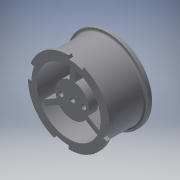
# Autodesk Inventor part: Wheel
Saved by Autodesk Inventor 2018 (Build 220112000, 112)
## iProperties
Created: 2018-12-29
Part Number: Wheel
Material: Типовые
Document SubType Name: Modeling
Designer: kostya
Density: 1 g/cm^3
Appearance: По умолчанию
Mass: 14.1359 g
Surface Area: 114.786 cm^2
Volume: 14.1359 cm^3
Author: kostya
Autodesk Inventor part; units mm, degrees
ref_plane "YZ Plane" through (0, 0, 0) normal (1, 0, 0) x (0, 1, 0)
ref_plane "XZ Plane" through (0, 0, 0) normal (0, 1, 0) x (-1, 0, 0)
ref_plane "XY Plane" through (0, 0, 0) normal (0, 0, 1) x (1, 0, 0)
sketch "Эскиз1" plane through (0, 0, 0) normal (0, 0, 1) x (1, 0, 0)
  line L0 (0, 0) -> (18, 0) construction
  line L1 (18, 0) -> (18, 24)
  line L2 (18, 24) -> (23, 24)
  line L3 (23, 0) -> (23, 24)
  line L4 (18, 0) -> (23, 0)
  line L5 (0, -4.8) -> (0, 28.8) projected
  line L6 (23, 0) -> (23, 2)
  line L7 (23, 2) -> (21, 2) construction
  line L8 (21, 3) -> (21, 18)
  line L9 (23, 24) -> (23, 22) construction
  line L10 (23, 22) -> (22, 22)
  line L11 (21, 21) -> (21, 18)
  arc A0 (22, 22) -> (21, 21) centre (22, 21) ccw
  line L12 (23, 12) -> (21, 12) construction
  arc A1 (21, 3) -> (22, 2) centre (22, 3) ccw
  line L13 (23, 2) -> (22, 2)
  point P0 (23, 18)
  dimension "d0" = 18
  dimension "d1" = 24
  dimension "d2" = 5
  dimension "d21" = 2
  dimension "d22" = 2
  dimension "d46" = 2
  constraints: 26 end point, 6 perpendicular, 4 point on circle, 4 point on line, 3 horizontal, 3 symmetric about line, 3 tangent, 2 centre point, 1 midpoint, 1 vertical, 1 other
  measures "d0" distance of L0.start L0.end
  measures "d1" distance of L0.end L1.end
  measures "d2" distance of L1.end L2.end
  measures "d21" distance of L3.start L6.end
  measures "d22" distance of L6.end L7.end
  measures "d46" distance of L2.end L9.end
revolve "Вращение1" add sketch "Эскиз1" angle 360 about axis through (0, -10, 0) along (0, 1, 0) contours L1 L2 L3 L10 A0 L11 L8 A1 L13 L4
ref_plane "РабПлоскость1" through (0, 12, 0) normal (0, 1, 0) x (1, 0, 0)
sketch "Эскиз5" plane through (0, 12, 0) normal (0, 1, 0) x (1, 0, 0)
  arc A0 (-1.0954, 0.95) -> (1.0954, 0.95) centre (0, 0) ccw
  line L0 (0.0475, -1.9475) -> (0.0475, 0.4525)
  line L1 (-1.0954, 0.95) -> (1.0954, 0.95)
  circle A1 centre (0, 0) radius 3
  circle A2 centre (0, 0) radius 18 projected
  circle A3 centre (0, 0) radius 18 projected
  line L2 (0.1379, -2.9968) -> (1.4256, -17.9435) construction
  line L3 (-1.0015, -2.8279) -> (-5.4596, -16.7697) construction
  line L4 (5.0855, 16.2079) -> (5.2328, 16.2079)
  line L5 (1.4256, 0.265) -> (1.4256, -0.265)
  line L6 (1.4256, -2.6396) -> (1.4256, -17.9435)
  line L7 (-1.4256, -17.9435) -> (-1.4256, -2.6396)
  line L8 (-1.4256, -0.265) -> (-1.4256, 0.265)
  arc A4 (-1.4256, -2.6396) -> (1.4256, -2.6396) centre (0, 0) ccw
  arc A5 (-1.4256, -17.9435) -> (1.4256, -17.9435) centre (0, -5.525) ccw
  dimension "d18" = 2.9
  dimension "d19" = 2.4
  dimension "d20" = 6
  constraints: 18 end point, 17 point on circle, 4 centre point, 4 parallel, 3 point on line, 2 coincident, 2 horizontal, 2 perpendicular, 1 concentric, 1 vertical, 2 other
  measures "d18" diameter of A0
  measures "d19" distance of L0.start L0.end
  measures "d20" diameter of A1
extrude "Выдавливание5" add sketch "Эскиз5" along normal mid plane 20 separate body contours A1 L6 A2 L7 | A2 A5 picked at (-0.6337, -12.9791)
pattern_circular "Круговой массив2" count 3 over 360 about axis through (0, -10, 0) along (0, 1, 0) of "Выдавливание5" bodies 2
extrude "Выдавливание6" add sketch "Эскиз5" along normal mid plane 20 contours A1 bodies 1
sketch "Эскиз6" plane through (0, 2, 0) normal (0, -1, 0) x (1, 0, 0)
  circle A0 centre (0, 0) radius 9.5
  arc A1 (1.0954, -0.95) -> (-1.0954, -0.95) centre (0, 0) ccw projected
  line L0 (1.0954, -0.95) -> (-1.0954, -0.95) projected
  dimension "d32" = 19
  constraints: 1 centre point, 1 coincident
  measures "d32" diameter of A0
extrude "Выдавливание7" add sketch "Эскиз6" against normal blind 5 bodies 1
sketch "Эскиз7" plane through (0, 2, 0) normal (0, -1, 0) x (1, 0, 0)
  circle A0 centre (0, 0) radius 9.5 projected
  arc A1 (1.0954, -0.95) -> (-1.0954, -0.95) centre (0, 0) ccw projected
  line L0 (1.0954, -0.95) -> (-1.0954, -0.95) projected
  arc A2 (1.0954, -0.95) -> (-1.0954, -0.95) centre (0, 0) ccw construction
  line L1 (0, 0) -> (-9.5, 0) construction
  line L2 (-1.45, 0) -> (-4.95, 0) construction
  line L3 (-4.95, 0) -> (-7.85, 0) construction
  circle A3 centre (-6.4, 0) radius 1.45
  line L4 (0, 0) -> (0, -9.5) construction
  circle A4 centre (0, -6.4) radius 1.45
  line L5 (0, 0) -> (9.5, 0) construction
  circle A5 centre (6.4, 0) radius 1.45
  line L6 (0, 0) -> (0, 9.5) construction
  circle A6 centre (0, 6.4) radius 1.45
  point P0 (0, -1.45)
  point P1 (0, -4.95)
  point P2 (0, -7.85)
  point P3 (1.45, 0)
  point P4 (4.95, 0)
  point P5 (7.85, 0)
  point P6 (0, 1.45)
  point P7 (0, 4.95)
  point P8 (0, 7.85)
  dimension "d35" = 3.5
  dimension "d36" = 2.9
  dimension "d39" = 360
  constraints: 12 end point, 12 point on line, 3 horizontal alignment, 2 vertical alignment, 1 horizontal, 1 midpoint, 1 point on circle, 42 other
  measures "d35" distance of L2.start L2.end
  measures "d36" distance of L2.end L3.end
extrude "Выдавливание8" cut sketch "Эскиз7" against normal up to next contours A3 | A5 bodies 1
sketch "Эскиз8" plane through (1.5732, 22, -2.5544) normal (0, 1, 0) x (0.8660254, 0, -0.5)
  circle A0 centre (2.9029, -4.6256) radius 1.45 projected
  circle A1 centre (2.9029, -4.6256) radius 2.5
  point P0 (-2.6396, -1.4256)
  dimension "d43" = 5
  constraints: 1 centre point, 1 coincident
  measures "d43" diameter of A1
extrude "Выдавливание9" cut sketch "Эскиз8" against normal up to next bodies 2
ref_plane "РабПлоскость3" through (0, 2, 17.9435) normal (-1, 0, 0) x (0, 0, 1)
mirror "Зеркальное отражение1" about plane through (0, 2, 17.9435) normal (-1, 0, 0) of "Выдавливание9" bodies 2
sketch "Эскиз9" plane through (0, 0, 0) normal (0, -1, 0) x (1, 0, 0)
  circle A0 centre (0, 0) radius 21 projected
  circle A1 centre (0, 0) radius 21 projected
  arc A2 (1.0954, -0.95) -> (-1.0954, -0.95) centre (0, 0) ccw projected
  circle A3 centre (0, 0) radius 23 projected
  circle A4 centre (0, 0) radius 23 projected
  arc A5 (-21.455, 8.2875) -> (-23, 0) centre (0, 0) ccw
  line L0 (-23, 0) -> (-21, 0)
  line L1 (-21.455, 8.2875) -> (-19.5151, 7.7563)
  constraints: 5 point on circle, 4 end point, 1 centre point, 1 coincident, 1 horizontal, 2 other
extrude "Выдавливание10" cut sketch "Эскиз9" against normal blind 10 contours A0 L0 A3 L1 picked at (-22.2755, 0.9397) bodies 1
pattern_circular "Круговой массив3" count 4 over 360 about axis through (0, 12, 0) along (0, 1, 0) of "Выдавливание10" bodies 1
